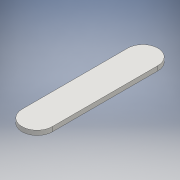
# Autodesk Inventor part: pads
Saved by Autodesk Inventor 2016 (Build 200138000, 138)
## iProperties
Created: 2016-02-20
Part Number: pads
Material: Generic
Document SubType Name: Modeling
Designer: Róbert
Density: 1 g/cm^3
Appearance: Default
Author: Róbert
Autodesk Inventor part; units mm, degrees
ref_plane "YZ Plane" through (0, 0, 0) normal (1, 0, 0) x (0, 1, 0)
ref_plane "XZ Plane" through (0, 0, 0) normal (0, 1, 0) x (-1, 0, 0)
ref_plane "XY Plane" through (0, 0, 0) normal (0, 0, 1) x (1, 0, 0)
sketch "Sketch1" plane through (0, 0, 0) normal (0, 0, 1) x (1, 0, 0)
  line L0 (0, 0) -> (0, 70)
  line L1 (20, 0) -> (20, 70)
  arc A0 (20, 70) -> (0, 70) centre (10, 70) ccw
  arc A1 (0, 0) -> (20, 0) centre (10, 0) ccw
  dimension "d1" = 70
  dimension "d3" = 70
  constraints: 4 end point, 4 point on circle, 3 tangent, 2 centre point, 2 vertical
  measures "d1" distance of L0.start L0.end
  measures "d3" distance of L1.start L1.end
extrude "Extrusion1" add sketch "Sketch1" along normal blind 3
body "Solid1"
